Autodesk Inventor part; units mm, degrees
(part 3 of 3)
  spline S29 degree 2 poles (-54.0032, 85.7381) (-52.5788, 85.7381) (-50.9733, 84.2314) (-50.9733, 82.947) knots 0 0 0 1 2 2 2
  spline S30 degree 2 poles (-50.9733, 82.947) (-50.9733, 82.346) (-51.2532, 81.3415) (-51.5002, 80.9134) knots 0 0 0 1 2 2 2
  spline S31 degree 2 poles (-51.5002, 80.9134) (-51.7472, 80.4688) (-52.4635, 79.596) (-52.8587, 79.1761) knots 0 0 0 1 2 2 2
  spline S32 degree 2 poles (-52.8587, 79.1761) (-53.5009, 78.4763) (-55.0735, 76.9778) (-55.5428, 76.5415) knots 0 0 0 1 2 2 2
  line L113 (-55.5428, 76.5415) -> (-50.5534, 76.5415)
  line L114 (-50.5534, 76.5415) -> (-50.5534, 75.3641)
  line L115 (-12.9466, 13.8805) -> (-6.681, 13.8805)
  line L116 (-6.681, 13.8805) -> (-6.681, 12.4397)
  spline S33 degree 2 poles (-6.681, 12.4397) (-7.3561, 11.8057) (-8.5582, 10.6283) (-9.1346, 9.9943) knots 0 0 0 1 2 2 2
  spline S34 degree 2 poles (-9.1346, 9.9943) (-10.2955, 8.7182) (-11.1435, 7.1868) (-11.1435, 6.3716) knots 0 0 0 1 2 2 2
  spline S35 degree 2 poles (-11.1435, 6.3716) (-11.1435, 5.9435) (-10.88, 5.3013) (-10.6413, 5.0955) knots 0 0 0 1 2 2 2
  spline S36 degree 2 poles (-10.6413, 5.0955) (-10.4025, 4.8896) (-9.7768, 4.6838) (-9.398, 4.6838) knots 0 0 0 1 2 2 2
  spline S37 degree 2 poles (-9.398, 4.6838) (-9.0358, 4.6838) (-8.2948, 4.8649) (-7.9572, 5.0049) knots 0 0 0 1 2 2 2
  spline S38 degree 2 poles (-7.9572, 5.0049) (-7.669, 5.1202) (-7.1338, 5.4495) (-6.9692, 5.5648) knots 0 0 0 1 2 2 2
  line L117 (-6.9692, 5.5648) -> (-6.8951, 5.5648)
  line L118 (-6.8951, 5.5648) -> (-6.8951, 4.1157)
  spline S39 degree 2 poles (-6.8951, 4.1157) (-7.315, 3.9099) (-8.8217, 3.5064) (-9.4968, 3.5064) knots 0 0 0 1 2 2 2
  spline S40 degree 2 poles (-9.4968, 3.5064) (-10.9212, 3.5064) (-12.5267, 5.0131) (-12.5267, 6.2975) knots 0 0 0 1 2 2 2
  spline S41 degree 2 poles (-12.5267, 6.2975) (-12.5267, 6.8986) (-12.2468, 7.9031) (-11.9998, 8.3312) knots 0 0 0 1 2 2 2
  spline S42 degree 2 poles (-11.9998, 8.3312) (-11.7528, 8.7758) (-11.0365, 9.6485) (-10.6413, 10.0684) knots 0 0 0 1 2 2 2
  spline S43 degree 2 poles (-10.6413, 10.0684) (-9.9991, 10.7683) (-8.4265, 12.2668) (-7.9572, 12.7031) knots 0 0 0 1 2 2 2
  line L119 (-7.9572, 12.7031) -> (-12.9466, 12.7031)
  line L120 (-12.9466, 12.7031) -> (-12.9466, 13.8805)
  point P0 (-25.6989, 67.7196)
  point P1 (-31.75, 68.8958)
  point P2 (-37.8011, 18.828)
  point P3 (-31.75, 20.0042)
  point P4 (-30.7426, 155.7595)
  point P5 (-31.75, 68.8958)
  point P6 (-31.75, 20.0009)
  point P7 (-53.7479, 68.8958)
  point P8 (-53.7479, 68.8958)
  point P9 (-9.7521, 20.0042)
  point P10 (-9.7521, 20.0042)
  point P11 (-25.5117, 69.1372)
  point P12 (-24.1982, 70.2173)
  point P13 (-24.4018, 70.4498)
  point P14 (-24.8053, 70.8498)
  point P15 (-25.2261, 71.2477)
  point P16 (-25.5299, 71.5084)
  point P17 (-26.7747, 72.3603)
  point P18 (-28.1162, 73.0109)
  point P19 (-29.5445, 73.4538)
  point P20 (-31.0399, 73.6839)
  point P21 (-31.4038, 73.7044)
  point P22 (-31.8144, 73.7105)
  point P23 (-32.2231, 73.7029)
  point P24 (-32.5832, 73.6811)
  point P25 (-34.1452, 73.4266)
  point P26 (-35.6245, 72.9413)
  point P27 (-37.023, 72.2212)
  point P28 (-38.2966, 71.2881)
  point P29 (-38.5728, 71.039)
  point P30 (-38.8889, 70.7308)
  point P31 (-39.1819, 70.4282)
  point P32 (-39.3698, 70.2107)
  point P33 (-38.0533, 69.1369)
  point P34 (-37.0798, 70.0849)
  point P35 (-35.9634, 70.8701)
  point P36 (-34.7501, 71.4605)
  point P37 (-33.4788, 71.8366)
  point P38 (-32.6411, 71.964)
  point P39 (-30.9237, 71.964)
  point P40 (-30.0858, 71.8365)
  point P41 (-28.8146, 71.461)
  point P42 (-27.6043, 70.8726)
  point P43 (-26.4919, 70.0903)
  point P44 (-27.4976, 67.2036)
  point P45 (-26.2023, 68.3104)
  point P46 (-26.2473, 68.3665)
  point P47 (-26.3703, 68.4988)
  point P48 (-26.5194, 68.6547)
  point P49 (-26.6838, 68.822)
  point P50 (-27.1503, 69.256)
  point P51 (-27.6238, 69.6269)
  point P52 (-28.1264, 69.9504)
  point P53 (-28.6869, 70.247)
  point P54 (-29.2441, 70.4848)
  point P55 (-29.83, 70.6775)
  point P56 (-30.433, 70.8217)
  point P57 (-31.0343, 70.9122)
  point P58 (-31.3562, 70.9333)
  point P59 (-31.8218, 70.939)
  point P60 (-32.2848, 70.9321)
  point P61 (-32.5832, 70.9098)
  point P62 (-33.5423, 70.7311)
  point P63 (-34.4536, 70.4349)
  point P64 (-35.3169, 70.0202)
  point P65 (-36.1406, 69.4848)
  point P66 (-36.4061, 69.2662)
  point P67 (-36.8094, 68.8887)
  point P68 (-37.2013, 68.5038)
  point P69 (-37.3635, 68.3097)
  point P70 (-36.0674, 67.2032)
  point P71 (-35.5544, 67.7509)
  point P72 (-34.9901, 68.2176)
  point P73 (-34.3779, 68.6001)
  point P74 (-33.7229, 68.8958)
  point P75 (-32.04, 69.2429)
  point P76 (-30.3491, 69.0602)
  point P77 (-28.7915, 68.36)
  point P78 (-29.4814, 65.242)
  point P79 (-29.4433, 65.1963)
  point P80 (-29.4105, 65.1624)
  point P81 (-29.3963, 65.1594)
  point P82 (-29.3562, 65.1846)
  point P83 (-28.7688, 65.736)
  point P84 (-28.1727, 66.2963)
  point P85 (-28.1634, 66.3178)
  point P86 (-28.1663, 66.3266)
  point P87 (-28.2084, 66.3834)
  point P88 (-28.258, 66.4485)
  point P89 (-28.3168, 66.5233)
  point P90 (-28.6224, 66.8616)
  point P91 (-28.9986, 67.1964)
  point P92 (-29.4081, 67.4984)
  point P93 (-29.8056, 67.7302)
  point P94 (-30.0613, 67.8432)
  point P95 (-30.3943, 67.9609)
  point P96 (-30.7335, 68.0617)
  point P97 (-31.0124, 68.1226)
  point P98 (-31.2629, 68.1554)
  point P99 (-31.5809, 68.1794)
  point P100 (-31.8907, 68.1916)
  point P101 (-32.0904, 68.184)
  point P102 (-32.8869, 68.0454)
  point P103 (-33.6094, 67.7947)
  point P104 (-34.263, 67.4283)
  point P105 (-34.8541, 66.9451)
  point P106 (-35.0435, 66.7537)
  point P107 (-35.2248, 66.5549)
  point P108 (-35.3825, 66.371)
  point P109 (-35.4014, 66.3193)
  point P110 (-35.3918, 66.297)
  point P111 (-34.7972, 65.7372)
  point P112 (-34.211, 65.1858)
  point P113 (-34.1695, 65.1598)
  point P114 (-34.1552, 65.163)
  point P115 (-34.1121, 65.2103)
  point P116 (-34.062, 65.2709)
  point P117 (-34.0071, 65.3446)
  point P118 (-33.6777, 65.7235)
  point P119 (-33.2792, 66.0389)
  point P120 (-32.8277, 66.2785)
  point P121 (-32.3411, 66.4325)
  point P122 (-32.0556, 66.4702)
  point P123 (-31.6858, 66.4725)
  point P124 (-31.3168, 66.4449)
  point P125 (-31.0333, 66.3878)
  point P126 (-30.6006, 66.2181)
  point P127 (-30.1846, 65.966)
  point P128 (-29.8154, 65.652)
  point P129 (-29.5219, 65.298)
  point P130 (-32.0702, 65.4015)
  point P131 (-32.1366, 65.3865)
  point P132 (-32.5528, 65.1937)
  point P133 (-32.8895, 64.8772)
  point P134 (-33.1084, 64.4743)
  point P135 (-33.1834, 64.0313)
  point P136 (-33.0397, 63.4202)
  point P137 (-32.6401, 62.9292)
  point P138 (-32.07, 62.6613)
  point P139 (-31.4495, 62.6738)
  point P140 (-31.0909, 62.817)
  point P141 (-30.7938, 63.0407)
  point P142 (-30.5702, 63.3378)
  point P143 (-30.4269, 63.6964)
  point P144 (-30.4151, 64.3239)
  point P145 (-30.6887, 64.8963)
  point P146 (-31.1898, 65.2927)
  point P147 (-31.8119, 65.4279)
  point P148 (-31.8933, 65.424)
  point P149 (-31.984, 65.4146)
  point P150 (-34.0186, 23.658)
  point P151 (-34.0567, 23.7037)
  point P152 (-34.0895, 23.7376)
  point P153 (-34.1037, 23.7406)
  point P154 (-34.1438, 23.7154)
  point P155 (-34.7312, 23.164)
  point P156 (-35.3273, 22.6037)
  point P157 (-35.3366, 22.5822)
  point P158 (-35.3337, 22.5734)
  point P159 (-35.2916, 22.5166)
  point P160 (-35.242, 22.4515)
  point P161 (-35.1832, 22.3767)
  point P162 (-34.8776, 22.0384)
  point P163 (-34.5014, 21.7036)
  point P164 (-34.0919, 21.4016)
  point P165 (-33.6944, 21.1698)
  point P166 (-33.4387, 21.0568)
  point P167 (-33.1057, 20.9391)
  point P168 (-32.7665, 20.8383)
  point P169 (-32.4876, 20.7774)
  point P170 (-32.2371, 20.7446)
  point P171 (-31.9191, 20.7206)
  point P172 (-31.6093, 20.7084)
  point P173 (-31.4096, 20.716)
  point P174 (-30.6131, 20.8546)
  point P175 (-29.8906, 21.1053)
  point P176 (-29.237, 21.4717)
  point P177 (-28.6459, 21.9549)
  point P178 (-28.4565, 22.1463)
  point P179 (-28.2752, 22.3451)
  point P180 (-28.1175, 22.529)
  point P181 (-28.0986, 22.5807)
  point P182 (-28.1082, 22.603)
  point P183 (-28.7028, 23.1628)
  point P184 (-29.289, 23.7142)
  point P185 (-29.3305, 23.7402)
  point P186 (-29.3448, 23.737)
  point P187 (-29.3879, 23.6897)
  point P188 (-29.438, 23.6291)
  point P189 (-29.4929, 23.5554)
  point P190 (-29.8223, 23.1765)
  point P191 (-30.2208, 22.8611)
  point P192 (-30.6723, 22.6215)
  point P193 (-31.1589, 22.4675)
  point P194 (-31.4444, 22.4298)
  point P195 (-31.8142, 22.4275)
  point P196 (-32.1832, 22.4551)
  point P197 (-32.4667, 22.5122)
  point P198 (-32.8994, 22.6819)
  point P199 (-33.3154, 22.934)
  dimension "d103" = 8.4153
  dimension "d105" = 0.508
  dimension "d106" = 0.508
  dimension "d107" = -2.9972
  dimension "d108" = 4.8735
  dimension "d110" = -4.8768
  dimension "d111" = 2.9972
  dimension "d112" = -2.9972
  constraints: 1360 point on circle, 680 centre point, 170 end point, 2 midpoint, 4 other
  measures "d103" distance of L12.end L14.start
  measures "d105" distance between parallel lines of L15 L7
  measures "d106" distance between parallel lines of L16 L11
  measures "d107" vertical distance of point (-30.743, 155.76) A129.centre
  measures "d108" vertical distance of point (-31.75, 68.896) A265.centre
  measures "d110" vertical distance of point (-31.75, 20.001) A401.centre
  measures "d111" vertical distance of point (-53.748, 68.896) A537.centre
  measures "d112" vertical distance of point (-9.752, 20.004) A673.centre
extrude "Extrusion20" add sketch "Sketch17" along normal blind 0.4 contours A167 A166 A165 A164 A163 A162 A161 A160 A159 A158 A157 A156 L40 L39 L38 L37 A155 A154 A153 A152 A151 A150 A149 A148 A147 A146 A145 A144 L36 L35 L34 L33 A143 A142 A141 A140 A139 A138 A137 A136 | A199 A198 A197 A196 A195 A194 A193 A192 A191 A190 A189 A188 A187 A186 A185 A184 L48 L47 L46 L45 A183 A182 A181 A180 A179 A178 A177 A176 L44 L43 L42 L41 A175 A174 A173 A172 A171 A170 A169 A168 | A251 A250 A249 A248 A247 A246 A245 A244 A243 A242 A241 A240 A239 A238 A237 A236 A235 A234 A233 A232 A231 A230 A229 A228 A227 A226 A225 A224 A223 A222 A221 A220 A219 A218 A217 A216 A215 A214 A213 A212 A211 A210 A209 A208 A207 A206 A205 A204 A203 A202 A201 A200 | A271 A270 A269 A268 A267 A266 A265 A264 A263 A262 A261 A260 A259 A258 A257 A256 A255 A254 A253 A252 | A303 A302 A301 A300 A299 A298 A297 A296 A295 A294 A293 A292 L56 L55 L54 L53 A291 A290 A289 A288 A287 A286 A285 A284 A283 A282 A281 A280 L52 L51 L50 L49 A279 A278 A277 A276 A275 A274 A273 A272 | A335 A334 A333 A332 A331 A330 A329 A328 A327 A326 A325 A324 A323 A322 A321 A320 L64 L63 L62 L61 A319 A318 A317 A316 A315 A314 A313 A312 L60 L59 L58 L57 A311 A310 A309 A308 A307 A306 A305 A304 | A387 A386 A385 A384 A383 A382 A381 A380 A379 A378 A377 A376 A375 A374 A373 A372 A371 A370 A369 A368 A367 A366 A365 A364 A363 A362 A361 A360 A359 A358 A357 A356 A355 A354 A353 A352 A351 A350 A349 A348 A347 A346 A345 A344 A343 A342 A341 A340 A339 A338 A337 A336 | A407 A406 A405 A404 A403 A402 A401 A400 A399 A398 A397 A396 A395 A394 A393 A392 A391 A390 A389 A388 | A439 A438 A437 A436 A435 A434 A433 A432 A431 A430 A429 A428 L72 L71 L70 L69 A427 A426 A425 A424 A423 A422 A421 A420 A419 A418 A417 A416 L68 L67 L66 L65 A415 A414 A413 A412 A411 A410 A409 A408 | A471 A470 A469 A468 A467 A466 A465 A464 A463 A462 A461 A460 A459 A458 A457 A456 L80 L79 L78 L77 A455 A454 A453 A452 A451 A450 A449 A448 L76 L75 L74 L73 A447 A446 A445 A444 A443 A442 A441 A440 | A523 A522 A521 A520 A519 A518 A517 A516 A515 A514 A513 A512 A511 A510 A509 A508 A507 A506 A505 A504 A503 A502 A501 A500 A499 A498 A497 A496 A495 A494 A493 A492 A491 A490 A489 A488 A487 A486 A485 A484 A483 A482 A481 A480 A479 A478 A477 A476 A475 A474 A473 A472 | A543 A542 A541 A540 A539 A538 A537 A536 A535 A534 A533 A532 A531 A530 A529 A528 A527 A526 A525 A524 | A575 A574 A573 A572 A571 A570 A569 A568 A567 A566 A565 A564 L88 L87 L86 L85 A563 A562 A561 A560 A559 A558 A557 A556 A555 A554 A553 A552 L84 L83 L82 L81 A551 A550 A549 A548 A547 A546 A545 A544 | A607 A606 A605 A604 A603 A602 A601 A600 A599 A598 A597 A596 A595 A594 A593 A592 L96 L95 L94 L93 A591 A590 A589 A588 A587 A586 A585 A584 L92 L91 L90 L89 A583 A582 A581 A580 A579 A578 A577 A576 | A659 A658 A657 A656 A655 A654 A653 A652 A651 A650 A649 A648 A647 A646 A645 A644 A643 A642 A641 A640 A639 A638 A637 A636 A635 A634 A633 A632 A631 A630 A629 A628 A627 A626 A625 A624 A623 A622 A621 A620 A619 A618 A617 A616 A615 A614 A613 A612 A611 A610 A609 A608 | A679 A678 A677 A676 A675 A674 A673 A672 A671 A670 A669 A668 A667 A666 A665 A664 A663 A662 A661 A660 | L97 L98 S0 S1 S2 S3 S4 S5 L99 L100 S6 S7 S8 S9 S10 L101 L102 | L103 L104 S11 S12 S13 S14 S15 S16 L105 L106 S17 S18 S19 S20 S21 L107 L108 bodies 2
sketch "Sketch18" plane through (0, 0, -0.2) normal (0, 0, -1) x (-1, 0, 0)
  line L0 (0, 0) -> (-63.5, 0)
  line L1 (-63.5, 0) -> (-63.5, 88.9)
  line L2 (-63.5, 88.9) -> (0, 88.9)
  line L3 (0, 88.9) -> (0, 0)
  constraints: 8 end point, 2 parallel, 1 horizontal, 1 perpendicular
extrude "Extrusion21" add sketch "Sketch18" along normal blind 0.4 bodies 3
fillet "Fillet2" radius 3.175 8 edges at (63.5, 0, 0.2) (63.5, 88.9, 0.2) (0, 0, 0.2) (0, 88.9, 0.2) (63.5, 0, -0.3) (63.5, 88.9, -0.3) (0, 0, -0.3) (0, 88.9, -0.3)
extrude "Extrusion22" cut sketch "Sketch17" along normal blind 0.4 contours A167 A166 A165 A164 A163 A162 A161 A160 A159 A158 A157 A156 L40 L39 L38 L37 A155 A154 A153 A152 A151 A150 A149 A148 A147 A146 A145 A144 L36 L35 L34 L33 A143 A142 A141 A140 A139 A138 A137 A136 | A199 A198 A197 A196 A195 A194 A193 A192 A191 A190 A189 A188 A187 A186 A185 A184 L48 L47 L46 L45 A183 A182 A181 A180 A179 A178 A177 A176 L44 L43 L42 L41 A175 A174 A173 A172 A171 A170 A169 A168 | A251 A250 A249 A248 A247 A246 A245 A244 A243 A242 A241 A240 A239 A238 A237 A236 A235 A234 A233 A232 A231 A230 A229 A228 A227 A226 A225 A224 A223 A222 A221 A220 A219 A218 A217 A216 A215 A214 A213 A212 A211 A210 A209 A208 A207 A206 A205 A204 A203 A202 A201 A200 | A271 A270 A269 A268 A267 A266 A265 A264 A263 A262 A261 A260 A259 A258 A257 A256 A255 A254 A253 A252 | A303 A302 A301 A300 A299 A298 A297 A296 A295 A294 A293 A292 L56 L55 L54 L53 A291 A290 A289 A288 A287 A286 A285 A284 A283 A282 A281 A280 L52 L51 L50 L49 A279 A278 A277 A276 A275 A274 A273 A272 | A335 A334 A333 A332 A331 A330 A329 A328 A327 A326 A325 A324 A323 A322 A321 A320 L64 L63 L62 L61 A319 A318 A317 A316 A315 A314 A313 A312 L60 L59 L58 L57 A311 A310 A309 A308 A307 A306 A305 A304 | A387 A386 A385 A384 A383 A382 A381 A380 A379 A378 A377 A376 A375 A374 A373 A372 A371 A370 A369 A368 A367 A366 A365 A364 A363 A362 A361 A360 A359 A358 A357 A356 A355 A354 A353 A352 A351 A350 A349 A348 A347 A346 A345 A344 A343 A342 A341 A340 A339 A338 A337 A336 | A407 A406 A405 A404 A403 A402 A401 A400 A399 A398 A397 A396 A395 A394 A393 A392 A391 A390 A389 A388 | A439 A438 A437 A436 A435 A434 A433 A432 A431 A430 A429 A428 L72 L71 L70 L69 A427 A426 A425 A424 A423 A422 A421 A420 A419 A418 A417 A416 L68 L67 L66 L65 A415 A414 A413 A412 A411 A410 A409 A408 | A471 A470 A469 A468 A467 A466 A465 A464 A463 A462 A461 A460 A459 A458 A457 A456 L80 L79 L78 L77 A455 A454 A453 A452 A451 A450 A449 A448 L76 L75 L74 L73 A447 A446 A445 A444 A443 A442 A441 A440 | A523 A522 A521 A520 A519 A518 A517 A516 A515 A514 A513 A512 A511 A510 A509 A508 A507 A506 A505 A504 A503 A502 A501 A500 A499 A498 A497 A496 A495 A494 A493 A492 A491 A490 A489 A488 A487 A486 A485 A484 A483 A482 A481 A480 A479 A478 A477 A476 A475 A474 A473 A472 | A543 A542 A541 A540 A539 A538 A537 A536 A535 A534 A533 A532 A531 A530 A529 A528 A527 A526 A525 A524 | A575 A574 A573 A572 A571 A570 A569 A568 A567 A566 A565 A564 L88 L87 L86 L85 A563 A562 A561 A560 A559 A558 A557 A556 A555 A554 A553 A552 L84 L83 L82 L81 A551 A550 A549 A548 A547 A546 A545 A544 | A607 A606 A605 A604 A603 A602 A601 A600 A599 A598 A597 A596 A595 A594 A593 A592 L96 L95 L94 L93 A591 A590 A589 A588 A587 A586 A585 A584 L92 L91 L90 L89 A583 A582 A581 A580 A579 A578 A577 A576 | A659 A658 A657 A656 A655 A654 A653 A652 A651 A650 A649 A648 A647 A646 A645 A644 A643 A642 A641 A640 A639 A638 A637 A636 A635 A634 A633 A632 A631 A630 A629 A628 A627 A626 A625 A624 A623 A622 A621 A620 A619 A618 A617 A616 A615 A614 A613 A612 A611 A610 A609 A608 | A679 A678 A677 A676 A675 A674 A673 A672 A671 A670 A669 A668 A667 A666 A665 A664 A663 A662 A661 A660 | L97 L98 S0 S1 S2 S3 S4 S5 L99 L100 S6 S7 S8 S9 S10 L101 L102 | L103 L104 S11 S12 S13 S14 S15 S16 L105 L106 S17 S18 S19 S20 S21 L107 L108 bodies 3
